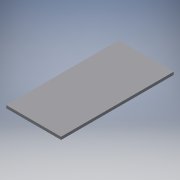
# Autodesk Inventor part: panel
Saved by Autodesk Inventor 2016 (Build 200138000, 138)
## iProperties
Created: 2017-06-12
Part Number: panel
Material: 一般
Document SubType Name: Modeling
Designer: B4_Ohno
Density: 1 g/cm^3
Appearance: 既定
Author: B4_Ohno
Autodesk Inventor part; units mm, degrees
ref_plane "YZ Plane" through (0, 0, 0) normal (1, 0, 0) x (0, 1, 0)
ref_plane "XZ Plane" through (0, 0, 0) normal (0, 1, 0) x (-1, 0, 0)
ref_plane "XY Plane" through (0, 0, 0) normal (0, 0, 1) x (1, 0, 0)
sketch "スケッチ1" plane through (0, 0, 0) normal (0, 0, 1) x (1, 0, 0)
  line L0 (-5.435, 14.9) -> (-5.435, -14.9) construction
  line L1 (-5.435, -14.9) -> (5.435, -14.9) construction
  line L2 (5.435, -14.9) -> (5.435, 14.9) construction
  line L3 (5.435, 14.9) -> (-5.435, 14.9) construction
  line L4 (9.065, 14.9) -> (-5.435, 14.9)
  line L5 (-5.435, 14.9) -> (-5.435, -14.9)
  line L6 (-5.435, -14.9) -> (9.065, -14.9)
  line L7 (9.065, -14.9) -> (9.065, 14.9)
  point P0 (0, 0)
  dimension "d0" = 14.5
  constraints: 8 end point, 2 parallel, 1 horizontal, 1 perpendicular
  measures "d0" distance of L0.end L6.end
extrude "押し出し1" add sketch "スケッチ1" along normal blind 0.725
